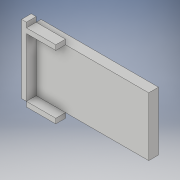
# Autodesk Inventor part: BackLiftProtoPart4
Saved by Autodesk Inventor 2017 (Build 210142000, 142)
## iProperties
Created: 2017-11-11
Part Number: BackLiftProtoPart4
Material: Generic
Document SubType Name: Modeling
Designer: User
Density: 1 g/cm^3
Appearance: Default
Author: User
Autodesk Inventor part; units mm, degrees
ref_plane "YZ Plane" through (0, 0, 0) normal (1, 0, 0) x (0, 1, 0)
ref_plane "XZ Plane" through (0, 0, 0) normal (0, 1, 0) x (-1, 0, 0)
ref_plane "XY Plane" through (0, 0, 0) normal (0, 0, 1) x (1, 0, 0)
sketch "Sketch1" plane through (0, 0, 0) normal (0, 0, 1) x (1, 0, 0)
  line L0 (0, 0) -> (304.8, 0)
  line L1 (304.8, 0) -> (304.8, 152.4)
  line L2 (304.8, 152.4) -> (0, 152.4)
  line L3 (0, 152.4) -> (0, 0)
  dimension "d0" = 304.8
  dimension "d1" = 152.4
  constraints: 8 end point, 2 parallel, 1 horizontal, 1 perpendicular
  measures "d0" distance of L2.end L1.end
  measures "d1" distance of L1.end L0.end
extrude "Extrusion1" add sketch "Sketch1" along normal blind 25.4
sketch "Sketch2" plane through (0, 0, 25.4) normal (0, 0, 1) x (1, 0, 0)
  line L0 (0, 0) -> (304.8, 0) projected
  line L1 (304.8, 152.4) -> (0, 152.4) projected
  line L2 (0, 0) -> (12.7, 0)
  line L3 (12.7, 0) -> (12.7, 152.4)
  line L4 (12.7, 152.4) -> (0, 152.4)
  line L5 (0, 152.4) -> (0, 0)
  dimension "d4" = 12.7
  constraints: 8 end point, 2 parallel, 1 horizontal, 1 perpendicular, 1 point on line
  measures "d4" distance of L4.end L3.end
extrude "Extrusion2" add sketch "Sketch2" along normal blind 25.4
sketch "Sketch3" plane through (0, 0, 0) normal (0, -1, 0) x (1, 0, 0)
  line L0 (304.8, 25.4) -> (12.7, 25.4) projected
  line L1 (12.7, 25.4) -> (88.9, 25.4)
  line L2 (88.9, 25.4) -> (88.9, 50.8)
  line L3 (88.9, 50.8) -> (12.7, 50.8)
  line L4 (12.7, 50.8) -> (12.7, 25.4)
  point P0 (0, 0)
  dimension "d7" = 76.2
  constraints: 8 end point, 2 parallel, 1 horizontal, 1 perpendicular
  measures "d7" distance of L3.end L2.end
sketch "Sketch4" plane through (0, 152.4, 0) normal (0, 1, 0) x (1, 0, 0)
  line L0 (304.8, -25.4) -> (12.7, -25.4) projected
  line L1 (12.7, -25.4) -> (88.9, -25.4)
  line L2 (88.9, -25.4) -> (88.9, -50.8)
  line L3 (88.9, -50.8) -> (12.7, -50.8)
  line L4 (12.7, -50.8) -> (12.7, -25.4)
  point P0 (0, 0)
  dimension "d8" = 76.2
  constraints: 8 end point, 2 parallel, 1 horizontal, 1 perpendicular
  measures "d8" distance of L2.end L3.end
extrude "Extrusion3" add sketch "Sketch4" along normal blind 12.7
extrude "Extrusion4" add sketch "Sketch3" along normal blind 12.7
sketch "Sketch5" plane through (12.7, 152.4, 25.4) normal (-1, 0, 0) x (0, 0, 1)
  point P0 (-25.4, -152.4)
sketch "Sketch6" plane through (0, 152.4, 0) normal (0, 1, 0) x (1, 0, 0)
  line L0 (12.7, -25.4) -> (12.7, -50.8) projected
  line L1 (0, 0) -> (0, -50.8) projected
  line L2 (12.7, -25.4) -> (0, -25.4)
  line L3 (0, -25.4) -> (0, -50.8)
  line L4 (0, -50.8) -> (12.7, -50.8)
  line L5 (12.7, -50.8) -> (12.7, -25.4)
  constraints: 8 end point, 2 parallel, 1 horizontal, 1 perpendicular
extrude "Extrusion5" add sketch "Sketch6" along normal blind 25.4
body "Solid1"
